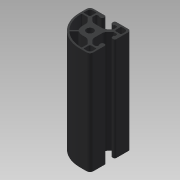
# Autodesk Inventor part: 40-4030-LITE-BLACK-FB
Saved by Autodesk Inventor 2013 (Build 170138000, 138)
## iProperties
Company: 80/20 Inc.
Created: 2014-04-23
Part Number: 40-4030-LITE-BLACK-FB
Material: Generic
Document SubType Name: Modeling
Designer: Ross Bowman
Density: 1 g/cm^3
Engineer: Ross Bowman
Catalog Web Link: 8020.net
Vendor: 80/20 Inc.
Material: 6105-T5 Aluminum
Author: Ross Bowman
Keywords: 80/20 , 8020 , T-Slot , Extrusion
Autodesk Inventor part; units mm, degrees
ref_plane "YZ Plane" through (0, 0, 0) normal (1, 0, 0) x (0, 1, 0)
ref_plane "XZ Plane" through (0, 0, 0) normal (0, 1, 0) x (-1, 0, 0)
ref_plane "XY Plane" through (0, 0, 0) normal (0, 0, 1) x (1, 0, 0)
sketch "Sketch1" plane through (0, 0, 0) normal (0, 0, 1) x (1, 0, 0)
  arc A0 (-8.8618, -11.1651) -> (9.517, -18.346) centre (10, 10) ccw
  arc A1 (-8.8935, -10.0603) -> (-8.8618, -11.1651) centre (-8.3561, -10.5977) ccw
  line L0 (-5.2779, -6.4446) -> (-8.8935, -10.0603)
  arc A2 (-4.3136, -6.3533) -> (-5.2779, -6.4446) centre (-4.7405, -6.982) ccw
  arc A3 (-4.3136, -6.3533) -> (0, -7.6793) centre (0, 0) ccw
  line L1 (3.3783, -7.6793) -> (0, -7.6793)
  arc A4 (6.7371, -9.0705) -> (3.3783, -7.6793) centre (3.3783, -12.4293) ccw
  line L2 (10.0673, -12.4008) -> (6.7371, -9.0705)
  arc A5 (10.2899, -12.9382) -> (10.0673, -12.4008) centre (9.5299, -12.9382) ccw
  line L3 (10.2899, -17.5861) -> (10.2899, -12.9382)
  arc A6 (9.517, -18.346) -> (10.2899, -17.5861) centre (9.5299, -17.5861) ccw
  line L4 (11.9399, -13.2101) -> (11.9399, -17.7201)
  arc A7 (13.2099, -11.9401) -> (11.9399, -13.2101) centre (13.2099, -13.2101) ccw
  line L5 (17.7199, -11.9401) -> (13.2099, -11.9401)
  arc A8 (18.3499, -12.5701) -> (17.7199, -11.9401) centre (17.7199, -12.5701) ccw
  line L6 (18.3499, -15.5501) -> (18.3499, -12.5701)
  arc A9 (15.5499, -18.3501) -> (18.3499, -15.5501) centre (15.5499, -15.5501) ccw
  line L7 (12.5699, -18.3501) -> (15.5499, -18.3501)
  arc A10 (11.9399, -17.7201) -> (12.5699, -18.3501) centre (12.5699, -17.7201) ccw
  line L8 (-11.9401, 13.2099) -> (-11.9401, 17.7199)
  arc A11 (-13.2101, 11.9399) -> (-11.9401, 13.2099) centre (-13.2101, 13.2099) ccw
  line L9 (-17.7201, 11.9399) -> (-13.2101, 11.9399)
  arc A12 (-18.3501, 12.5699) -> (-17.7201, 11.9399) centre (-17.7201, 12.5699) ccw
  line L10 (-18.3501, 15.5499) -> (-18.3501, 12.5699)
  arc A13 (-15.5501, 18.3499) -> (-18.3501, 15.5499) centre (-15.5501, 15.5499) ccw
  line L11 (-12.5701, 18.3499) -> (-15.5501, 18.3499)
  arc A14 (-11.9401, 17.7199) -> (-12.5701, 18.3499) centre (-12.5701, 17.7199) ccw
  line L12 (-9.0705, 6.7371) -> (-12.4008, 10.0673)
  arc A15 (-7.6793, 3.3783) -> (-9.0705, 6.7371) centre (-12.4293, 3.3783) ccw
  line L13 (-7.6793, 0) -> (-7.6793, 3.3783)
  arc A16 (-7.6793, 0) -> (-6.3533, -4.3136) centre (0, 0) ccw
  arc A17 (-6.4446, -5.2779) -> (-6.3533, -4.3136) centre (-6.982, -4.7405) ccw
  line L14 (-10.0603, -8.8935) -> (-6.4446, -5.2779)
  arc A18 (-11.1651, -8.8618) -> (-10.0603, -8.8935) centre (-10.5977, -8.3561) ccw
  arc A19 (-18.346, 9.517) -> (-11.1651, -8.8618) centre (10, 10) ccw
  arc A20 (-17.5861, 10.2899) -> (-18.346, 9.517) centre (-17.5861, 9.5299) ccw
  line L15 (-12.9382, 10.2899) -> (-17.5861, 10.2899)
  arc A21 (-12.4008, 10.0673) -> (-12.9382, 10.2899) centre (-12.9382, 9.5299) ccw
  circle A22 centre (0, 0) radius 3.4
  line L16 (13.195, 11.925) -> (17.705, 11.925)
  arc A23 (11.925, 13.195) -> (13.195, 11.925) centre (13.195, 13.195) ccw
  line L17 (11.925, 17.705) -> (11.925, 13.195)
  arc A24 (12.555, 18.335) -> (11.925, 17.705) centre (12.555, 17.705) ccw
  line L18 (15.535, 18.335) -> (12.555, 18.335)
  arc A25 (18.335, 15.535) -> (15.535, 18.335) centre (15.535, 15.535) ccw
  line L19 (18.335, 12.555) -> (18.335, 15.535)
  arc A26 (17.705, 11.925) -> (18.335, 12.555) centre (17.705, 12.555) ccw
  arc A27 (20, 17.1424) -> (17.1424, 20) centre (17.1424, 17.1424) ccw
  line L20 (17.1424, 20) -> (5.5403, 20)
  arc A28 (5.5403, 20) -> (4.06, 18.5197) centre (5.5403, 18.5197) ccw
  line L21 (4.06, 18.5197) -> (4.06, 17.8048)
  arc A29 (4.06, 17.8048) -> (5.9248, 15.94) centre (5.9248, 17.8048) ccw
  line L22 (5.9248, 15.94) -> (7.2807, 15.94)
  line L23 (7.2807, 15.94) -> (7.2807, 16.7)
  line L24 (7.2807, 16.7) -> (9.015, 16.7)
  arc A30 (10.285, 15.43) -> (9.015, 16.7) centre (9.015, 15.43) ccw
  line L25 (10.285, 15.43) -> (10.285, 13.0538)
  arc A31 (9.9772, 12.3106) -> (10.285, 13.0538) centre (9.234, 13.0538) ccw
  line L26 (9.9772, 12.3106) -> (7.0978, 9.4312)
  arc A32 (3.739, 8.04) -> (7.0978, 9.4312) centre (3.739, 12.79) ccw
  line L27 (3.739, 8.04) -> (-3.739, 8.04)
  arc A33 (-7.0978, 9.4312) -> (-3.739, 8.04) centre (-3.739, 12.79) ccw
  line L28 (-7.0978, 9.4312) -> (-10.0243, 12.3578)
  arc A34 (-10.285, 12.9871) -> (-10.0243, 12.3578) centre (-9.395, 12.9871) ccw
  line L29 (-10.285, 12.9871) -> (-10.285, 15.3633)
  arc A35 (-8.9483, 16.7) -> (-10.285, 15.3633) centre (-8.9483, 15.3633) ccw
  line L30 (-8.9483, 16.7) -> (-7.2807, 16.7)
  line L31 (-7.2807, 16.7) -> (-7.2807, 15.94)
  line L32 (-7.2807, 15.94) -> (-5.9248, 15.94)
  arc A36 (-5.9248, 15.94) -> (-4.06, 17.8048) centre (-5.9248, 17.8048) ccw
  line L33 (-4.06, 17.8048) -> (-4.06, 18.5197)
  arc A37 (-4.06, 18.5197) -> (-5.5403, 20) centre (-5.5403, 18.5197) ccw
  line L34 (-5.5403, 20) -> (-16.833, 20)
  arc A38 (-16.833, 20) -> (-20, 16.833) centre (-16.833, 16.833) ccw
  line L35 (-20, 16.833) -> (-20, 10)
  arc A39 (-20, 10) -> (10, -20) centre (10, 10) ccw
  line L36 (10, -20) -> (16.833, -20)
  arc A40 (16.833, -20) -> (20, -16.833) centre (16.833, -16.833) ccw
  line L37 (20, -16.833) -> (20, -5.5403)
  arc A41 (20, -5.5403) -> (18.5197, -4.06) centre (18.5197, -5.5403) ccw
  line L38 (18.5197, -4.06) -> (17.8048, -4.06)
  arc A42 (17.8048, -4.06) -> (15.94, -5.9248) centre (17.8048, -5.9248) ccw
  line L39 (15.94, -5.9248) -> (15.94, -7.2807)
  line L40 (15.94, -7.2807) -> (16.7, -7.2807)
  line L41 (16.7, -7.2807) -> (16.7, -8.9483)
  arc A43 (15.3633, -10.285) -> (16.7, -8.9483) centre (15.3633, -8.9483) ccw
  line L42 (15.3633, -10.285) -> (12.9871, -10.285)
  arc A44 (12.3578, -10.0243) -> (12.9871, -10.285) centre (12.9871, -9.395) ccw
  line L43 (12.3578, -10.0243) -> (9.4312, -7.0978)
  arc A45 (8.04, -3.739) -> (9.4312, -7.0978) centre (12.79, -3.739) ccw
  line L44 (8.04, -3.739) -> (8.04, 3.739)
  arc A46 (9.4312, 7.0978) -> (8.04, 3.739) centre (12.79, 3.739) ccw
  line L45 (9.4312, 7.0978) -> (12.3106, 9.9772)
  arc A47 (13.0538, 10.285) -> (12.3106, 9.9772) centre (13.0538, 9.234) ccw
  line L46 (13.0538, 10.285) -> (15.43, 10.285)
  arc A48 (16.7, 9.015) -> (15.43, 10.285) centre (15.43, 9.015) ccw
  line L47 (16.7, 9.015) -> (16.7, 7.2807)
  line L48 (16.7, 7.2807) -> (15.94, 7.2807)
  line L49 (15.94, 7.2807) -> (15.94, 5.9248)
  arc A49 (15.94, 5.9248) -> (17.8048, 4.06) centre (17.8048, 5.9248) ccw
  line L50 (17.8048, 4.06) -> (18.5197, 4.06)
  arc A50 (18.5197, 4.06) -> (20, 5.5403) centre (18.5197, 5.5403) ccw
  line L51 (20, 5.5403) -> (20, 17.1424)
  constraints: 104 end point, 100 point on circle, 51 centre point
extrude "Extrusion1" add sketch "Sketch1" against normal blind 100
body "Solid1"
